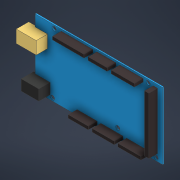
# Autodesk Inventor part: ArduinoMega
Saved by Autodesk Inventor 2021 (Build 250183000, 183)
## iProperties
Created: 2020-12-16
Part Number: ArduinoMega
Material: Generisch
Document SubType Name: Modeling
Designer: laure
Density: 1 g/cm^3
Appearance: Vorgabe
Author: laure
Autodesk Inventor part; units mm, degrees
ref_plane "YZ Plane" through (0, 0, 0) normal (1, 0, 0) x (0, 1, 0)
ref_plane "XZ Plane" through (0, 0, 0) normal (0, 1, 0) x (-1, 0, 0)
ref_plane "XY Plane" through (0, 0, 0) normal (0, 0, 1) x (1, 0, 0)
sketch "Skizze1" plane through (0, 0, 0) normal (0, 0, 1) x (1, 0, 0)
  line L0 (-50.8, 26.67) -> (50.8, 26.67)
  line L1 (50.8, 26.67) -> (50.8, -26.67)
  line L2 (50.8, -26.67) -> (-50.8, -26.67)
  line L3 (-50.8, -26.67) -> (-50.8, 26.67)
  line L4 (0, -37.338) -> (0, 37.338) projected
  line L5 (-78.32, 0) -> (72.32, 0) projected
  circle A0 centre (-35.56, 24.13) radius 1.6
  circle A1 centre (-36.83, -24.13) radius 1.6
  circle A2 centre (39.37, 24.13) radius 1.6
  circle A3 centre (45.72, -24.13) radius 1.6
  circle A4 centre (15.24, -19.05) radius 1.6
  line L6 (-29.812, 25.1729) -> (-4.812, 25.1729)
  line L7 (-4.812, 25.1729) -> (-4.812, 22.67)
  line L8 (-4.812, 22.67) -> (-29.812, 22.67)
  line L9 (-29.812, 22.67) -> (-29.812, 25.1729)
  line L10 (-1.4087, 25.1729) -> (13.5913, 25.1729)
  line L11 (13.5913, 25.1729) -> (13.5913, 22.6729)
  line L12 (13.5913, 22.6729) -> (-1.4087, 22.6729)
  line L13 (-1.4087, 22.6729) -> (-1.4087, 25.1729)
  line L14 (16.84, 25.1729) -> (35.34, 25.1729)
  line L15 (35.34, 25.1729) -> (35.34, 22.6729)
  line L16 (35.34, 22.6729) -> (16.84, 22.6729)
  line L17 (16.84, 22.6729) -> (16.84, 25.1729)
  line L18 (46.87, 24.13) -> (43.37, 24.13)
  line L19 (43.37, 24.13) -> (43.37, -20.87)
  line L20 (43.37, -20.87) -> (46.87, -20.87)
  line L21 (46.87, -20.87) -> (46.87, 24.13)
  line L22 (40.4611, -25.17) -> (22.2148, -25.17)
  line L23 (22.2148, -25.17) -> (22.2148, -22.67)
  line L24 (22.2148, -22.67) -> (40.4611, -22.67)
  line L25 (40.4611, -22.67) -> (40.4611, -25.17)
  line L26 (19.229, -22.67) -> (1.6551, -22.67)
  line L27 (1.6551, -22.67) -> (1.6551, -25.17)
  line L28 (1.6551, -25.17) -> (19.229, -25.17)
  line L29 (19.229, -25.17) -> (19.229, -22.67)
  line L30 (-1.4087, -22.67) -> (-17.312, -22.67)
  line L31 (-17.312, -22.67) -> (-17.312, -25.17)
  line L32 (-17.312, -25.17) -> (-1.4087, -25.17)
  line L33 (-1.4087, -25.17) -> (-1.4087, -22.67)
  line L34 (-56.8, 17.67) -> (-40.8, 17.67)
  line L35 (-40.8, 17.67) -> (-40.8, 7.67)
  line L36 (-40.8, 7.67) -> (-56.8, 7.67)
  line L37 (-56.8, 7.67) -> (-56.8, 17.67)
  line L38 (-52.8, -14.67) -> (-38.8, -14.67)
  line L39 (-38.8, -14.67) -> (-38.8, -23.17)
  line L40 (-38.8, -23.17) -> (-52.8, -23.17)
  line L41 (-52.8, -23.17) -> (-52.8, -14.67)
  point P0 (0, 0)
  point P1 (-50.8, 17.67)
  point P2 (-50.8, 7.67)
  point P3 (-50.8, -14.67)
  point P4 (-50.8, -23.17)
  dimension "d0" = 101.6
  dimension "d1" = 53.34
  dimension "d2" = 3.2
  dimension "d3" = 15.24
  dimension "d4" = 3.2
  dimension "d5" = 13.97
  dimension "d6" = 2.54
  dimension "d7" = 48.26
  dimension "d8" = 3.2
  dimension "d9" = 90.17
  dimension "d10" = 3.2
  dimension "d11" = 96.52
  dimension "d12" = 3.2
  dimension "d13" = 66.04
  dimension "d14" = 7.62
  dimension "d15" = 25
  dimension "d16" = 4
  dimension "d17" = 15
  dimension "d18" = 2.5
  dimension "d19" = 18.5
  dimension "d20" = 3.5
  dimension "d21" = 45
  dimension "d22" = 4
  dimension "d23" = 2.5
  dimension "d24" = 4
  dimension "d25" = 9
  dimension "d26" = 10
  dimension "d27" = 16
  dimension "d28" = 6
  dimension "d29" = 8.5
  dimension "d30" = 3.5
  dimension "d31" = 14
  dimension "d32" = 2
  constraints: 80 end point, 20 parallel, 10 horizontal, 10 perpendicular, 5 centre point, 5 point on line, 2 other
  measures "d0" distance between parallel lines of L1 L3
  measures "d1" distance between parallel lines of L0 L2
  measures "d2" diameter of A0
  measures "d3" distance from line of L3 A0.centre
  measures "d4" diameter of A1
  measures "d5" distance from line of L3 A1.centre
  measures "d6" distance from line of L2 A1.centre
  measures "d7" vertical distance of A0.centre A1.centre
  measures "d8" diameter of A2
  measures "d9" distance from line of L3 A2.centre
  measures "d10" diameter of A3
  measures "d11" distance from line of L3 A3.centre
  measures "d12" diameter of A4
  measures "d13" distance from line of L3 A4.centre
  measures "d14" distance from line of L2 A4.centre
  measures "d15" distance between parallel lines of L9 L7
  measures "d16" distance between parallel lines of L0 L8
  measures "d17" distance of L11.end L12.end
  measures "d18" distance of L10.end L11.end
  measures "d19" distance of L15.end L16.end
  measures "d20" distance of L20.end L19.end
  measures "d21" distance of L19.end L18.end
  measures "d22" distance from line of L19 A2.centre
  measures "d23" distance of L22.end L23.end
  measures "d24" distance between parallel lines of L2 L30
  measures "d25" distance between parallel lines of L34 L0
  measures "d26" distance between parallel lines of L36 L34
  measures "d27" distance between parallel lines of L35 L37
  measures "d28" distance between parallel lines of L3 L37
  measures "d29" distance between parallel lines of L40 L38
  measures "d30" distance between parallel lines of L40 L2
  measures "d31" distance between parallel lines of L39 L41
  measures "d32" distance between parallel lines of L41 L3
extrude "Extrusion1" add sketch "Skizze1" along normal blind 1 contours L0 L4 L10 L13 L12 L5 L3 L36 L35 L34 | L0 L1 L5 L21 L18 L19 L4 L12 L11 L10 | L1 L2 L4 L5 L19 L20 L21 | L5 L4 L2 L3 L40 L39 L38
extrude "Extrusion2" add sketch "Skizze1" along normal blind 8 contours L10 L11 L12 L4 | L4 L12 L13 L10 | L6 L7 L8 L9 | L14 L15 L16 L17 | L22 L23 L24 L25 | L29 L28 L27 L26 | L33 L32 L31 L30
extrude "Extrusion3" add sketch "Skizze1" along normal blind 8 contours L21 L20 L19 L5 | L5 L19 L18 L21
extrude "Extrusion5" add sketch "Skizze1" along normal blind 10 contours L34 L35 L36 L3 | L3 L36 L37 L34
extrude "Extrusion6" add sketch "Skizze1" along normal blind 10 contours L38 L39 L40 L3 | L3 L40 L41 L38
